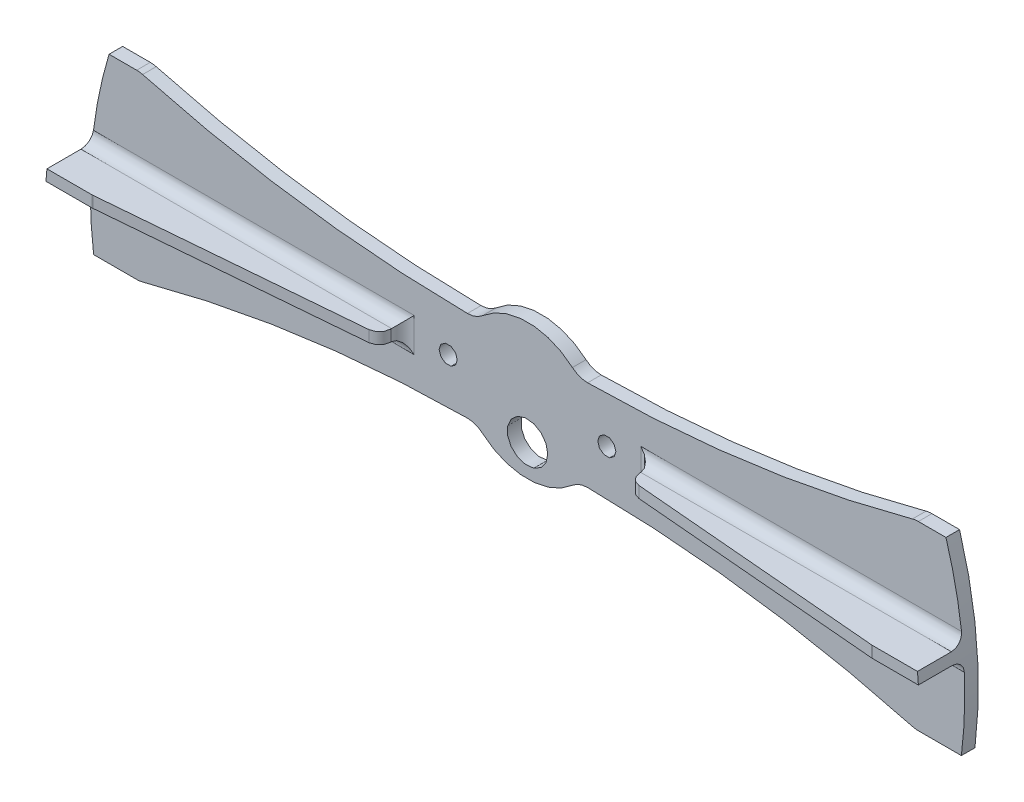
# Autodesk Inventor part: Schrittmotor aufnahme
Saved by Autodesk Inventor 2023 (Build 270158000, 158)
## iProperties
Created: 2026-03-17
Part Number: Schrittmotor aufnahme
Material: Generisch
Document SubType Name: Modeling
Designer: lerat
Density: 1 g/cm^3
Appearance: Vorgabe
Author: lerat
Autodesk Inventor part; units mm, degrees
ref_plane "YZ Plane" through (0, 0, 0) normal (1, 0, 0) x (0, 1, 0)
ref_plane "XZ Plane" through (0, 0, 0) normal (0, 1, 0) x (-1, 0, 0)
ref_plane "XY Plane" through (0, 0, 0) normal (0, 0, 1) x (1, 0, 0)
sketch "Skizze1" plane through (0, 0, 0) normal (0, 0, 1) x (1, 0, 0)
  spline S0 degree 3 poles (99.5, 0.0001) (99.5003, 3.5138) (99.3162, 7.008) (98.9479, 10.4823) (98.2325, 17.2318) (96.8181, 23.9219) (94.7421, 30.3976) (93.7264, 33.5661) (92.5531, 36.6803) (91.2275, 39.7252) (89.9242, 42.7189) (88.4734, 45.6463) (86.8814, 48.4968) (85.3162, 51.2994) (83.6145, 54.0277) (81.7844, 56.6691) (79.985, 59.266) (78.0616, 61.7785) (76.0226, 64.1941) (74.0178, 66.5692) (71.9012, 68.8505) (69.6814, 71.028) (67.499, 73.1689) (65.2169, 75.2094) (62.8457, 77.1405) (60.5144, 79.0391) (58.0972, 80.8319) (55.6061, 82.5109) (53.1568, 84.1616) (50.6362, 85.7023) (48.054, 87.1271) (43.0375, 89.8951) (37.7862, 92.2254) (32.3614, 94.0903) (29.707, 95.0028) (27.0115, 95.8039) (24.2864, 96.4899) (18.9925, 97.8227) (13.5902, 98.7189) (8.1588, 99.1654) (2.9077, 99.5972) (-2.3733, 99.6111) (-7.6276, 99.2073) (-10.1986, 99.0098) (-12.7632, 98.7121) (-15.3137, 98.3148) (-20.2686, 97.5428) (-25.1702, 96.3936) (-29.9496, 94.8854) (-32.2882, 94.1475) (-34.5976, 93.3239) (-36.8722, 92.4166) (-41.2911, 90.6541) (-45.5795, 88.5751) (-49.7017, 86.1974) (-53.687, 83.8987) (-57.5173, 81.3207) (-61.1529, 78.4889) (-64.6678, 75.751) (-67.9995, 72.7762) (-71.1159, 69.5914) (-74.1288, 66.5124) (-76.941, 63.2365) (-79.5289, 59.7937) (-82.0309, 56.4652) (-84.3231, 52.9815) (-86.3869, 49.3718) (-88.3822, 45.8819) (-90.1642, 42.2739) (-91.7219, 38.5683) (-93.228, 34.9858) (-94.5248, 31.3111) (-95.6034, 27.5703) (-96.6462, 23.9538) (-97.4845, 20.2765) (-98.1113, 16.5671) (-98.7173, 12.9809) (-99.1256, 9.3646) (-99.3349, 5.7378) (-99.5371, 2.2315) (-99.5536, -1.2852) (-99.3843, -4.7953) (-99.2206, -8.189) (-98.883, -11.5766) (-98.3721, -14.9402) (-97.8782, -18.1921) (-97.2222, -21.4214) (-96.4088, -24.6081) (-95.6223, -27.689) (-94.689, -30.7295) (-93.614, -33.7151) (-92.5748, -36.6016) (-91.403, -39.4374) (-90.1024, -42.2132) (-88.8451, -44.8968) (-87.4674, -47.5243) (-85.9741, -50.0869) (-84.5304, -52.5644) (-82.9786, -54.9813) (-81.3241, -57.3285) (-79.7245, -59.5977) (-78.0289, -61.8016) (-76.2439, -63.9308) (-72.8341, -67.9981) (-69.0982, -71.7909) (-65.0877, -75.2589) (-61.3404, -78.4994) (-57.3524, -81.4579) (-53.1671, -84.1039) (-51.1879, -85.3552) (-49.1647, -86.5366) (-47.1021, -87.6452) (-43.1619, -89.7631) (-39.0771, -91.6155) (-34.8824, -93.1853) (-30.9628, -94.6522) (-26.9477, -95.872) (-22.8776, -96.8338) (-20.9529, -97.2887) (-19.0158, -97.686) (-17.0699, -98.0251) (-13.3527, -98.6729) (-9.6028, -99.1083) (-5.8387, -99.3292) (-2.3217, -99.5357) (1.2078, -99.5549) (4.7305, -99.3871) (8.022, -99.2302) (11.3075, -98.91) (14.5697, -98.4275) (20.5926, -97.5367) (26.5364, -96.0905) (32.2986, -94.1122) (37.3139, -92.3904) (42.191, -90.2667) (46.8649, -87.7717) (50.9329, -85.6001) (54.8468, -83.1475) (58.5736, -80.4334) (61.8173, -78.0712) (64.92, -75.5101) (67.8583, -72.7698) (70.4157, -70.3847) (72.8479, -67.8646) (75.139, -65.2257) (79.0792, -60.6876) (82.6006, -55.7985) (85.6551, -50.6306) (87.9272, -46.7864) (89.942, -42.7872) (91.6803, -38.6656) (92.9733, -35.5998) (94.1131, -32.4662) (95.0928, -29.2842) (96.5327, -24.6075) (97.626, -19.8302) (98.362, -15.009) (99.0803, -10.3041) (99.4591, -5.5561) (99.4969, -0.7675) knots 0 0 0 0 0.016785 0.016785 0.016785 0.049393 0.049393 0.049393 0.065348 0.065348 0.065348 0.081035 0.081035 0.081035 0.096458 0.096458 0.096458 0.111622 0.111622 0.111622 0.126531 0.126531 0.126531 0.14119 0.14119 0.14119 0.155602 0.155602 0.155602 0.169773 0.169773 0.169773 0.1973 0.1973 0.1973 0.21077 0.21077 0.21077 0.236936 0.236936 0.236936 0.262234 0.262234 0.262234 0.274612 0.274612 0.274612 0.298658 0.298658 0.298658 0.310424 0.310424 0.310424 0.333281 0.333281 0.333281 0.35538 0.35538 0.35538 0.376744 0.376744 0.376744 0.397399 0.397399 0.397399 0.417368 0.417368 0.417368 0.436675 0.436675 0.436675 0.45534 0.45534 0.45534 0.473385 0.473385 0.473385 0.490831 0.490831 0.490831 0.507698 0.507698 0.507698 0.524004 0.524004 0.524004 0.53977 0.53977 0.53977 0.555011 0.555011 0.555011 0.569747 0.569747 0.569747 0.583993 0.583993 0.583993 0.597766 0.597766 0.597766 0.611082 0.611082 0.611082 0.636519 0.636519 0.636519 0.660287 0.660287 0.660287 0.671527 0.671527 0.671527 0.692998 0.692998 0.692998 0.71306 0.71306 0.71306 0.722548 0.722548 0.722548 0.740671 0.740671 0.740671 0.757606 0.757606 0.757606 0.773429 0.773429 0.773429 0.802643 0.802643 0.802643 0.828069 0.828069 0.828069 0.850199 0.850199 0.850199 0.86946 0.86946 0.86946 0.886225 0.886225 0.886225 0.915055 0.915055 0.915055 0.9365 0.9365 0.9365 0.952453 0.952453 0.952453 0.975899 0.975899 0.975899 0.998779 0.998779 0.998779 0.998779 projected
  circle A0 centre (-17.5, 8) radius 2 projected
  circle A1 centre (17.5, 8) radius 2 projected
  circle A2 centre (0, 0) radius 4.4663 projected
  arc A3 (-9.3133, 18.4126) -> (-10.9526, 16.6718) centre (0, 8) ccw projected
  arc A4 (-9.9152, -3.2556) -> (0, -7) centre (0, 8) ccw
  arc A5 (-92.3485, 28) -> (-95.751, -12) centre (0, 0) ccw
  line L0 (-95.751, -12) -> (-92.3485, 28) construction
  line L1 (-95.751, -12) -> (-86.251, -12) construction
  arc A6 (-13.2571, -2.0077) -> (-84.9421, -11.8257) centre (-11.1803, -283.78) ccw
  line L2 (-11.1803, -2) -> (-36.6655, -2) construction
  line L3 (0, 8) -> (-94.0498, 8) construction
  line L4 (-95.751, 28) -> (-85.582, 28) construction
  arc A7 (-84.9421, 27.8257) -> (-13.2571, 18.0077) centre (-11.1803, 299.78) ccw
  line L5 (-92.3485, 28) -> (-85.582, 28) construction
  line L6 (-92.3485, 28) -> (-86.251, 28)
  line L7 (-95.751, -12) -> (-86.251, -12)
  arc A8 (-86.251, -12) -> (-84.9421, -11.8257) centre (-86.251, -7) ccw
  arc A9 (-84.9421, 27.8257) -> (-86.251, 28) centre (-86.251, 23) ccw
  arc A10 (-15, 8) -> (-11.1803, -2) centre (0, 8) ccw construction
  arc A11 (-11.1803, 18) -> (-15, 8) centre (0, 8) ccw construction
  arc A12 (-9.9152, -3.2556) -> (-13.2571, -2.0077) centre (-13.2202, -7.0075) ccw
  arc A13 (-13.2571, 18.0077) -> (-9.9152, 19.2556) centre (-13.2202, 23.0075) ccw
  line L8 (0, 23) -> (0, -7) construction
  arc A14 (0, -7) -> (0, 23) centre (0, 8) ccw construction
  arc A15 (0, 23) -> (-9.9152, 19.2556) centre (0, 8) ccw
  circle A16 centre (17.5, 8) radius 2
  arc A17 (10.9526, 16.6718) -> (9.3133, 18.4126) centre (0, 8) ccw
  arc A18 (0, -7) -> (9.9152, -3.2556) centre (0, 8) ccw
  arc A19 (95.751, -12) -> (92.3485, 28) centre (0, 0) ccw
  line L9 (95.751, -12) -> (86.251, -12) construction
  arc A20 (84.9421, -11.8257) -> (13.2571, -2.0077) centre (11.1803, -283.78) ccw
  line L10 (11.1803, -2) -> (36.6655, -2) construction
  line L11 (0, 8) -> (94.0498, 8) construction
  arc A21 (13.2571, 18.0077) -> (84.9421, 27.8257) centre (11.1803, 299.78) ccw
  line L12 (95.751, 28) -> (85.582, 28) construction
  line L13 (92.3485, 28) -> (85.582, 28) construction
  line L14 (92.3485, 28) -> (86.251, 28)
  line L15 (95.751, -12) -> (86.251, -12)
  arc A22 (84.9421, -11.8257) -> (86.251, -12) centre (86.251, -7) ccw
  arc A23 (86.251, 28) -> (84.9421, 27.8257) centre (86.251, 23) ccw
  arc A24 (11.1803, -2) -> (15, 8) centre (0, 8) ccw construction
  arc A25 (15, 8) -> (11.1803, 18) centre (0, 8) ccw construction
  arc A26 (13.2571, -2.0077) -> (9.9152, -3.2556) centre (13.2202, -7.0075) ccw
  arc A27 (9.9152, 19.2556) -> (13.2571, 18.0077) centre (13.2202, 23.0075) ccw
  arc A28 (9.9152, 19.2556) -> (0, 23) centre (0, 8) ccw
  dimension "d0" = 30
  dimension "d1" = 96.5
  dimension "d2" = 40
  dimension "d4" = 10
  dimension "d5" = 5
  dimension "d6" = 9.5
  dimension "d7" = 5
  dimension "d8" = 5
  constraints: 60 point on circle, 32 end point, 29 symmetric about line, 25 centre point, 9 tangent, 4 horizontal, 4 point on line, 3 coincident, 2 collinear, 2 midpoint, 1 equal radius, 1 horizontal alignment, 1 vertical, 1 vertical alignment, 14 other
  measures "d0" diameter of A4
  measures "d1" radius of A5
  measures "d2" vertical distance of L0.start L0.end
  measures "d4" distance from line of A0.centre L2
  measures "d5" radius of A8
  measures "d6" horizontal distance of L0.start A8.centre
  measures "d7" radius of A12
  measures "d8" radius of A13
extrude "Extrusion1" add sketch "Skizze1" against normal blind 3
sketch "Skizze2" plane through (0, 0, 0) normal (0, 0, 1) x (1, 0, 0)
  arc A0 (-9.9152, -3.2556) -> (9.9152, -3.2556) centre (0, 8) ccw projected
  arc A1 (13.2571, -2.0077) -> (9.9152, -3.2556) centre (13.2202, -7.0075) ccw projected
  arc A2 (84.9421, -11.8257) -> (13.2571, -2.0077) centre (11.1803, -283.78) ccw projected
  arc A3 (84.9421, -11.8257) -> (86.251, -12) centre (86.251, -7) ccw projected
  line L0 (86.251, -12) -> (95.751, -12) projected
  arc A4 (95.751, -12) -> (92.3485, 28) centre (0, 0) ccw projected
  line L1 (92.3485, 28) -> (86.251, 28) projected
  arc A5 (86.251, 28) -> (84.9421, 27.8257) centre (86.251, 23) ccw projected
  arc A6 (13.2571, 18.0077) -> (84.9421, 27.8257) centre (11.1803, 299.78) ccw projected
  arc A7 (9.9152, 19.2556) -> (13.2571, 18.0077) centre (13.2202, 23.0075) ccw projected
  arc A8 (9.9152, 19.2556) -> (-9.9152, 19.2556) centre (0, 8) ccw projected
  arc A9 (-13.2571, 18.0077) -> (-9.9152, 19.2556) centre (-13.2202, 23.0075) ccw projected
  arc A10 (-84.9421, 27.8257) -> (-13.2571, 18.0077) centre (-11.1803, 299.78) ccw projected
  arc A11 (-84.9421, 27.8257) -> (-86.251, 28) centre (-86.251, 23) ccw projected
  line L2 (-86.251, 28) -> (-92.3485, 28) projected
  arc A12 (-92.3485, 28) -> (-95.751, -12) centre (0, 0) ccw projected
  line L3 (-95.751, -12) -> (-86.251, -12) projected
  arc A13 (-86.251, -12) -> (-84.9421, -11.8257) centre (-86.251, -7) ccw projected
  arc A14 (-13.2571, -2.0077) -> (-84.9421, -11.8257) centre (-11.1803, -283.78) ccw projected
  arc A15 (-9.9152, -3.2556) -> (-13.2571, -2.0077) centre (-13.2202, -7.0075) ccw projected
  circle A16 centre (17.5, 8) radius 2 projected
  circle A17 centre (0, 0) radius 4.4663 projected
  circle A18 centre (-17.5, 8) radius 2 projected
  arc A19 (-92.3485, 28) -> (-95.751, -12) centre (0, 0) ccw projected
  line L4 (-96.0556, 9.25) -> (-27.5, 9.25)
  line L5 (-27.5, 9.25) -> (-27.5, 6.75)
  line L6 (-27.5, 6.75) -> (-96.2636, 6.75)
  point P0 (-27.5, 8)
  point P1 (-96.0556, 9.25)
  point P2 (-96.2636, 6.75)
  dimension "d11" = 2.5
  dimension "d12" = 10
  constraints: 6 end point, 2 horizontal, 2 point on circle, 1 horizontal alignment, 1 midpoint, 1 vertical
  measures "d11" distance of L4.end L5.end
  measures "d12" distance from line of A18.centre L5
extrude "Extrusion2" add sketch "Skizze2" along normal blind 10 contours A12 L4 L5 L6
sketch "Skizze3" plane through (-96.0556, 9.25, 0) normal (0, 1, 0) x (1, 0, 0)
  line L0 (68.5556, -10) -> (0, -10) projected
  line L1 (10, -10) -> (68.5556, -5)
  line L2 (68.5556, 0) -> (68.5556, -10) projected
  line L3 (82.7986, 0) -> (11.1135, 0) projected
  line L4 (0, 0) -> (0, -10) projected
  point P0 (96.0556, 0)
  dimension "d15" = 5
  dimension "d16" = 10
  constraints: 2 end point, 1 midpoint, 1 point on line
  measures "d15" distance from line of L1.end L3
  measures "d16" distance from line of L1.start L4
extrude "Extrusion3" cut sketch "Skizze3" against normal blind 10
fillet "Rundung1" radius 2.5 4 edges at (-27.5, 8, 5) (-86.0556, 8, 10) (-61.7778, 9.25, 0) (-61.8818, 6.75, 0)
fillet "Rundung2" radius 2.5 3 edges at (-27.5, 10.5, 0) (-27.5, 8, 0) (-27.5, 5.5, 0)
mirror "Spiegeln1" about plane through (0, 0, 0) normal (1, 0, 0) of "Extrusion2", "Extrusion3", "Rundung1", "Rundung2"
